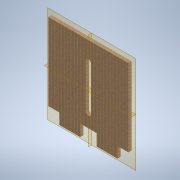
# Autodesk Inventor part: Hammer_wall
Saved by Autodesk Inventor 2021 (Build 250183000, 183)
## iProperties
Created: 2021-02-17
Part Number: Hammer_wall
Material: MDF Medium Density Fiberboard
Document SubType Name: Modeling
Designer: negt20
Density: 0.8 g/cm^3
Appearance: Cardboard - Corrugated
Author: negt20
Autodesk Inventor part; units mm, degrees
sketch "Sketch1" plane through (0, 0, 0) normal (0, 0, 1) x (1, 0, 0)
  line L0 (-73.5, 80.75) -> (73.5, 80.75)
  line L1 (73.5, 80.75) -> (73.5, -80.75)
  line L2 (73.5, -80.75) -> (-73.5, -80.75)
  line L3 (-73.5, -80.75) -> (-73.5, 80.75)
  point P0 (0, 80.75)
  point P1 (0, 0)
  point P2 (-73.5, 0)
  dimension "d0" = 147
  dimension "d1" = 161.5
  constraints: 8 end point, 2 midpoint, 2 parallel, 1 horizontal, 1 horizontal alignment, 1 perpendicular, 1 vertical alignment
  measures "d0" distance of L1.end L2.end
  measures "d1" distance of L0.end L1.end
extrude "Extrusion1" add sketch "Sketch1" along normal blind 6
sketch "Sketch2" plane through (0, 0, 6) normal (0, 0, 1) x (1, 0, 0)
  line L0 (-73.5, 80.75) -> (-73.5, -80.75) projected
  line L1 (-73.5, -80.75) -> (-73.5, -60.75)
  line L2 (-53.5, -80.75) -> (-73.5, -80.75)
  line L3 (-73.5, -60.75) -> (-53.5, -60.75)
  line L4 (-53.5, -60.75) -> (-53.5, -80.75)
  line L5 (-73.5, -80.75) -> (73.5, -80.75) projected
  line L6 (-53.5, -80.75) -> (-73.5, -80.75)
  point P0 (0, 0)
  point P1 (40.5, -62.5)
  dimension "d14" = 20
  dimension "d18" = 20
  constraints: 10 end point, 1 collinear, 1 horizontal, 1 perpendicular, 1 point on line
  measures "d14" distance of L0.end L1.end
  measures "d18" distance of L1.end L3.end
extrude "Extrusion2" cut sketch "Sketch2" against normal blind 15
mirror "Mirror1" about plane through (0, 0, 0) normal (1, 0, 0) of "Extrusion2"
sketch "Sketch5" plane through (0, 0, 6) normal (0, 0, 1) x (1, 0, 0)
  line L0 (-15, -59.25) -> (15, -59.25)
  line L1 (15, -59.25) -> (15, -80.75)
  line L2 (15, -80.75) -> (-15, -80.75)
  line L3 (-15, -80.75) -> (-15, -59.25)
  line L4 (-53.5, -80.75) -> (53.5, -80.75) projected
  point P0 (0, 0)
  point P1 (0, -80.75)
  point P2 (0, -80.75)
  point P3 (0, -80.75)
  dimension "d19" = 30
  dimension "d20" = 21.5
  constraints: 8 end point, 3 midpoint, 2 coincident, 2 parallel, 1 horizontal, 1 perpendicular
  measures "d19" distance of L1.end L2.end
  measures "d20" distance of L0.end L1.end
extrude "Extrusion4" cut sketch "Sketch5" against normal blind 6
sketch "Sketch3" plane through (0, 0, 6) normal (0, 0, 1) x (1, 0, 0)
  line L0 (-73.5, -80.75) -> (73.5, -80.75) projected
  line L1 (-15, -59.25) -> (15, -59.25) projected
  line L2 (0, -80.75) -> (0, -69.25) construction
  line L3 (0, -69.25) -> (0, -44.25) construction
  line L4 (0, -44.25) -> (0, -34.25) construction
  line L5 (-5, 45.75) -> (5, 45.75) construction
  line L6 (5, 45.75) -> (5, -34.25)
  line L7 (5, -34.25) -> (-5, -34.25) construction
  line L8 (-5, -34.25) -> (-5, 45.75)
  arc A0 (-5, -34.25) -> (5, -34.25) centre (0, -34.25) ccw
  arc A1 (5, 45.75) -> (-5, 45.75) centre (0, 45.75) ccw
  line L9 (73.5, 80.75) -> (-73.5, 80.75) projected
  line L10 (0, 80.75) -> (0, 55.75) construction
  line L11 (0, 55.75) -> (0, 45.75) construction
  point P0 (0, 0)
  point P1 (-40.5, -62.5)
  point P2 (40.5, -62.5)
  point P3 (73.5, -80.75)
  dimension "d23" = 11.5
  dimension "d24" = 25
  dimension "d26" = 10
  dimension "d27" = 10
  dimension "d29" = 25
  dimension "d30" = 10
  constraints: 18 end point, 4 point on circle, 3 midpoint, 3 vertical, 2 centre point, 2 parallel, 1 coincident, 1 horizontal, 1 perpendicular, 1 point on line, 2 other
  measures "d23" distance of L2.start L2.end
  measures "d24" distance of L3.end L2.end
  measures "d26" distance of L4.end L3.end
  measures "d27" distance of L6.end L7.end
  measures "d29" distance of L10.start L10.end
  measures "d30" distance of L11.end L10.end
extrude "Extrusion3" cut sketch "Sketch3" against normal blind 6
equation "\"d7\" = d5"
equation "\"d5\" = 15"
body "Solid1"
